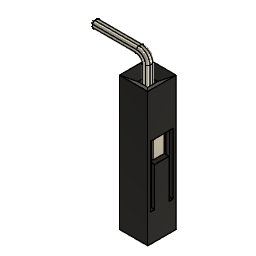
Male_90 (Autodesk Fusion 360 design; units mm, degrees)
Autodesk Fusion 360 part; units mm, degrees
note: some values were not read from the file. Set by a fixed rule: which sketch regions a step uses.
sketch "Sketch1" plane through (0, 0, 0) normal (0, 0, 1) x (1, 0, 0)
  line L0 (1.27, -1.27) -> (-1.27, -1.27)
  line L1 (-1.27, -1.27) -> (-1.27, 1.27)
  line L2 (-1.27, 1.27) -> (1.27, 1.27)
  line L3 (1.27, 1.27) -> (1.27, -1.27)
  line L4 (1.27, -1.27) -> (-1.27, 1.27) construction
  line L5 (-1.27, -1.27) -> (1.27, 1.27) construction
  dimension "d1" = 2.54
  dimension "d2" = 2.54
  constraint horizontal L0
  constraint perpendicular L0 L1
  constraint parallel L0 L2
  constraint parallel L1 L3
  constraint coincident L4 origin
  constraint coincident L5 origin
  measures "d1" distance of L1.end L2.end
  measures "d2" distance of L0.end L1.end
extrude "Extrude1" add sketch "Sketch1" along normal blind 12
sketch "Sketch2" plane through (0, 0, 12) normal (0, 0, 1) x (-1, 0, 0)
  line L0 (-1.27, -1.27) -> (1.27, -1.27)
  line L1 (1.27, -1.27) -> (1.27, 1.27)
  line L2 (1.27, 1.27) -> (-1.27, 1.27)
  line L3 (-1.27, 1.27) -> (-1.27, -1.27)
  line L4 (-0.45, 0.45) -> (0.45, 0.45)
  line L5 (0.45, 0.45) -> (0.45, -0.45)
  line L6 (0.45, -0.45) -> (-0.45, -0.45)
  line L7 (-0.45, -0.45) -> (-0.45, 0.45)
  line L8 (-0.45, 0.45) -> (0.45, -0.45) construction
  line L9 (0.45, 0.45) -> (-0.45, -0.45) construction
  dimension "d5" = 0.9
  dimension "d6" = 0.9
  constraint horizontal L4
  constraint perpendicular L4 L5
  constraint parallel L4 L6
  constraint parallel L5 L7
  constraint coincident L8 origin
  constraint coincident L9 origin
  measures "d5" distance of L5.end L6.end
  measures "d6" distance of L4.end L5.end
extrude "Extrude2" cut sketch "Sketch2" against normal blind 0.5 contours L4 L5 L6 L7
loft "Loft1" cut profiles "Sketch2" section 1 section 2 face at (0.15, -0.15, 11.5)
extrude "Extrude3" cut 1 faces at (0.15, -0.15, 11.5) along direction (0, 0, -1) blind 8
sketch "Sketch3" plane through (1.27, 0, 0) normal (1, 0, 0) x (0, 1, 0)
  line L0 (-1.27, 0) -> (1.27, 0)
  line L1 (1.27, 0) -> (1.27, 12)
  line L2 (1.27, 12) -> (-1.27, 12)
  line L3 (-1.27, 12) -> (-1.27, 0)
  line L4 (1, 8) -> (-1, 8)
  line L5 (-1, 8) -> (-1, 2.5)
  line L6 (-1, 2.5) -> (1, 2.5)
  line L7 (1, 2.5) -> (1, 8)
  line L8 (1, 8) -> (-1, 2.5) construction
  line L9 (-1, 8) -> (1, 2.5) construction
  line L10 (0.6482, 2.5061) -> (-0.6518, 2.5061)
  line L11 (-0.6518, 2.5061) -> (-0.6518, 6.0061)
  line L12 (-0.6518, 6.0061) -> (0.6482, 6.0061)
  line L13 (0.6482, 6.0061) -> (0.6482, 2.5061)
  line L14 (0.6482, 2.5061) -> (-0.6518, 6.0061) construction
  line L15 (-0.6518, 2.5061) -> (0.6482, 6.0061) construction
  line L16 (-0.6518, 6.0061) -> (0.6571, 6.0061)
  line L17 (0.6571, 6.0061) -> (0.6571, 8.0061)
  line L18 (0.6571, 8.0061) -> (-0.6518, 8.0061)
  line L19 (-0.6518, 8.0061) -> (-0.6518, 6.0061)
  line L20 (0.5, 6.1311) -> (-0.5, 6.1311)
  line L21 (-0.5, 6.1311) -> (-0.5, 7.8811)
  line L22 (-0.5, 7.8811) -> (0.5, 7.8811)
  line L23 (0.5, 7.8811) -> (0.5, 6.1311)
  line L24 (0.5, 6.1311) -> (-0.5, 7.8811) construction
  line L25 (-0.5, 6.1311) -> (0.5, 7.8811) construction
  line L26 (-1.27, 6) -> (-0.6518, 6.0061)
  line L27 (0.6571, 6.0061) -> (1.27, 6)
  line L28 (0.6482, 2.5061) -> (1, 2.5)
  line L29 (-0.6518, 2.5061) -> (-1, 2.5)
  point P0 (0, 5.25)
  point P1 (-0.0018, 4.2561)
  point P2 (0, 7.0061)
  dimension "d11" = 5.5
  dimension "d12" = 2.5
  dimension "d13" = 1.3
  dimension "d14" = 3.5
  dimension "d15" = 2
  dimension "d16" = 1
  dimension "d17" = 1.75
  dimension "d31" = 0.125
  constraint horizontal L4
  constraint perpendicular L4 L5
  constraint parallel L4 L6
  constraint parallel L5 L7
  constraint coincident L8 P0
  constraint coincident L9 P0
  constraint horizontal L10
  constraint perpendicular L10 L11
  constraint parallel L10 L12
  constraint parallel L11 L13
  constraint coincident L14 P1
  constraint coincident L15 P1
  constraint horizontal L16
  constraint vertical L17
  constraint horizontal L18
  constraint vertical L19
  constraint horizontal L20
  constraint perpendicular L20 L21
  constraint parallel L20 L22
  constraint parallel L21 L23
  constraint coincident L24 P2
  constraint coincident L25 P2
  constraint midpoint L3 L26.start
  constraint midpoint L1 L27.end
  measures "d11" distance of L4.end L5.end
  measures "d12" distance of L0 L6
  measures "d13" distance of L11.end L12.end
  measures "d14" distance of L10.end L11.end
  measures "d15" distance of L11.end L18.end
  measures "d16" distance of L21.end L22.end
  measures "d17" distance of L20.end L21.end
  measures "d31" distance of L18 L22
extrude "Extrude4" cut sketch "Sketch3" against normal blind 0.3 contours L5 L11 L26 L29 | L4 L5 L19 L26 | L4 L7 L17 L27 | L7 L13 L16 L27 L28
extrude "Extrude5" cut sketch "Sketch3" against normal blind 0.5 contours L4 L12 L16 L17 L19
extrude "Extrude6" cut sketch "Sketch3" against normal blind 0.3 contours L20 L21 L22 L23
sketch "Sketch4" plane through (0, 0, 0) normal (0, 0, -1) x (1, 0, 0)
  line L0 (-1.27, -1.27) -> (1.27, -1.27)
  line L1 (1.27, -1.27) -> (1.27, 1.27)
  line L2 (1.27, 1.27) -> (-1.27, 1.27)
  line L3 (-1.27, 1.27) -> (-1.27, -1.27)
  line L4 (0.75, -0.75) -> (-0.75, -0.75)
  line L5 (-0.75, -0.75) -> (-0.75, 0.75)
  line L6 (-0.75, 0.75) -> (0.75, 0.75)
  line L7 (0.75, 0.75) -> (0.75, -0.75)
  line L8 (0.75, -0.75) -> (-0.75, 0.75) construction
  line L9 (-0.75, -0.75) -> (0.75, 0.75) construction
  dimension "d24" = 1.5
  dimension "d25" = 1.5
  constraint horizontal L4
  constraint perpendicular L4 L5
  constraint parallel L4 L6
  constraint parallel L5 L7
  constraint coincident L8 origin
  constraint coincident L9 origin
  measures "d24" distance of L5.end L6.end
  measures "d25" distance of L4.end L5.end
extrude "Extrude7" cut sketch "Sketch4" against normal blind 2 contours L4 L5 L6 L7
sketch "Sketch5" plane through (0, 0, 2) normal (0, 0, -1) x (1, 0, 0)
  line L0 (0.75, 0.75) -> (-0.75, 0.75)
  line L1 (-0.75, 0.75) -> (-0.75, -0.75)
  line L2 (-0.75, -0.75) -> (0.75, -0.75)
  line L3 (0.75, -0.75) -> (0.75, 0.75)
  circle A0 centre (0, 0) radius 0.725
  dimension "d28" = 1.45
  constraint coincident A0.centre origin
  measures "d28" diameter of A0
extrude "Extrude8" add sketch "Sketch5" along normal blind 0.1 contours A0
sketch "Sketch6" plane through (0, 0, 3.5) normal (0, 0, 1) x (-1, 0, 0)
  line L0 (-0.45, -0.45) -> (0.45, -0.45)
  line L1 (0.45, -0.45) -> (0.45, 0.45)
  line L2 (0.45, 0.45) -> (-0.45, 0.45)
  line L3 (-0.45, 0.45) -> (-0.45, -0.45)
  line L4 (-0.325, 0.325) -> (0.325, 0.325)
  line L5 (0.325, 0.325) -> (0.325, -0.325)
  line L6 (0.325, -0.325) -> (-0.325, -0.325)
  line L7 (-0.325, -0.325) -> (-0.325, 0.325)
  line L8 (-0.325, 0.325) -> (0.325, -0.325) construction
  line L9 (0.325, 0.325) -> (-0.325, -0.325) construction
  dimension "d32" = 0.65
  dimension "d33" = 0.65
  constraint horizontal L4
  constraint perpendicular L4 L5
  constraint parallel L4 L6
  constraint parallel L5 L7
  constraint coincident L8 origin
  constraint coincident L9 origin
  measures "d32" distance of L5.end L6.end
  measures "d33" distance of L4.end L5.end
extrude "Extrude9" add sketch "Sketch6" along normal blind 10.5 contours L4 L5 L6 L7
sketch "Sketch7" plane through (-0.325, 0, 0) normal (-1, 0, 0) x (0, -1, 0)
  line L0 (-0.325, 3.5) -> (0.325, 3.5)
  line L1 (0.325, 3.5) -> (0.325, 14)
  line L2 (0.325, 14) -> (-0.325, 14)
  line L3 (-0.325, 14) -> (-0.325, 3.5)
  line L4 (-0.325, 14) -> (0.325, 14)
  line L5 (0.325, 14) -> (0.325, 13.35)
  line L6 (0.325, 13.35) -> (-0.325, 13.35)
  line L7 (-0.325, 13.35) -> (-0.325, 14)
  dimension "d38" = 0.65
  constraint horizontal L4
  constraint vertical L5
  constraint horizontal L6
  constraint vertical L7
  constraint coincident L2.end L3.start
  constraint coincident L1.end L5
  measures "d38" distance of L2.end L6.end
extrude "Extrude10" add sketch "Sketch7" along normal blind 4.5 contours L1 L2 L3 L4 L5 L6 L7
fillet "Fillet1" radius 0.2 12 edges at (0.325, -0.325, 8.75) (-0.325, -0.325, 8.425) (0.325, 0.325, 8.75) (-0.325, 0.325, 8.425) (-2.25, 0.325, 14) (-2.25, -0.325, 14) (-2.575, -0.325, 13.35) (-2.575, 0.325, 13.35) (-4.825, -0.325, 13.675) (-4.825, 0.325, 13.675) (-4.825, 0, 14) (-4.825, 0, 13.35)
fillet "Fillet1" radius 1 1 edges at (0.325, 0, 14)
fillet "Fillet1" radius 0.5 1 edges at (-0.325, 0, 13.35)
equation "d34 = 8.50 mm + 2 mm"
named bodies: "Male_90"
